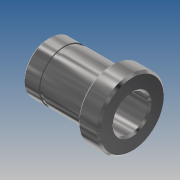
# Autodesk Inventor part: DD_KVD_004_03
Saved by Autodesk Inventor 2017.3 (Build 213256000, 256)
## iProperties
Created: 2012-08-17
Part Number: DD_KVD_004_03
Material: Nerezová ocel
Document SubType Name: Modeling
Designer: DAŘENA M.
Manufacturer: Standard
Standards Organization: Custom
Mass: 243.623 g
Surface Area: 187.558 cm^2
Volume: 30.4529 cm^3
Density: 8 g/cm^3
Appearance: Pololeštěná
HRUBA_HMOTNOST: 1,18 kg
POLOTOVAR_NORMA: ČSN 425510
ROZMER_POLOTOVARU: KR 80 - 30
Title: HRŘÍEL KLADKY
Author: DAŘENA M.
Autodesk Inventor part; units mm, degrees
ref_plane "YZ Plane" through (0, 0, 0) normal (1, 0, 0) x (0, 1, 0)
ref_plane "XZ Plane" through (0, 0, 0) normal (0, 1, 0) x (-1, 0, 0)
ref_plane "XY Plane" through (0, 0, 0) normal (0, 0, 1) x (1, 0, 0)
sketch "Náčrt1" plane through (0, 0, 0) normal (0, 0, 1) x (1, 0, 0)
  line L0 (-8, 0) -> (8, 0)
  line L1 (8, 0) -> (8, 27.5) construction
  line L2 (8, 27.5) -> (5.5, 27.5) construction
  line L3 (5.5, 27.5) -> (5.5, 26.5) construction
  line L4 (0.5, 21.5) -> (-0.5, 21.5) construction
  line L5 (-5.5, 26.5) -> (-5.5, 27.5) construction
  line L6 (-5.5, 27.5) -> (-8, 27.5) construction
  line L7 (-8, 27.5) -> (-8, 0) construction
  line L8 (-8, 16) -> (-6.85, 16) construction
  line L9 (-6.85, 16) -> (-6.85, 17.25) construction
  line L10 (-6.85, 17.25) -> (-5, 17.25) construction
  line L11 (-5, 17.25) -> (-5, 16) construction
  line L12 (-5, 16) -> (5, 16) construction
  line L13 (5, 16) -> (5, 14) construction
  line L14 (5, 14) -> (8, 14) construction
  arc A0 (-5.5, 26.5) -> (-0.5, 21.5) centre (-0.5, 26.5) ccw construction
  arc A1 (0.5, 21.5) -> (5.5, 26.5) centre (0.5, 26.5) ccw construction
  line L15 (5, 6) -> (5, 8)
  line L16 (5, 8) -> (10, 8)
  line L17 (10, 8) -> (10, 0)
  line L18 (10, 0) -> (8, 0)
  line L19 (-10, 6) -> (-10, 0)
  line L20 (-10, 0) -> (-8, 0)
  line L21 (-5, 6) -> (-5, 5.75)
  line L22 (-5, 5.75) -> (-6.1, 5.75)
  line L23 (-6.1, 5.75) -> (-6.1, 6)
  line L24 (-5, 6) -> (5, 6)
  line L25 (-6.1, 6) -> (-10, 6)
  point P0 (0, 0)
  point P1 (0, 0)
  point P2 (5.5, 21.5)
  point P3 (-5.5, 21.5)
  dimension "d0" = 55
  dimension "d1" = 16
  dimension "d3" = 2.5
  dimension "d4" = 6
  dimension "d5" = 32
  dimension "d6" = 28
  dimension "d7" = 10
  dimension "d8" = 13
  dimension "d9" = 34.5
  dimension "d10" = 1.85
  dimension "d18" = 11
  dimension "d24" = 43
  dimension "d27" = 5
  dimension "d31" = 16
  dimension "d32" = 2
  dimension "d33" = 2
  dimension "d34" = 1.1
  dimension "d35" = 11.5
  dimension "d36" = 12
  dimension "d37" = 20
  constraints: 52 end point, 10 horizontal, 9 vertical, 6 collinear, 6 perpendicular, 6 point on line, 4 point on circle, 4 tangent, 2 centre point, 2 coincident, 1 equal radius, 1 midpoint
  measures "d0" diameter of L1.end L0
  measures "d1" distance between parallel lines of L1 L7
  measures "d3" distance of L5.end L6.end
  measures "d4" distance of point (-5.5, 21.5) L5.end
  measures "d5" diameter of L12 L0
  measures "d6" diameter of L14 L0
  measures "d7" distance of L11.end L12.end
  measures "d8" distance from line of L7 L13.end
  measures "d9" diameter of L10 L0
  measures "d10" distance of L9.end L10.end
  measures "d18" distance of point (5.5, 21.5) point (-5.5, 21.5)
  measures "d24" diameter of L4 L0
  measures "d27" radius of A0
  measures "d31" diameter of L16 L0
  measures "d32" distance between parallel lines of L17 L1
  measures "d33" distance between parallel lines of L7 L19
  measures "d34" distance of L21.end L22.end
  measures "d35" diameter of L22 L0
  measures "d36" diameter of L25 L20
  measures "d37" distance between parallel lines of L17 L19
revolve "Rotace1" add sketch "Náčrt1" angle 360 about axis through (-8, 0, 0) along (1, 0, 0)
chamfer "Zkosení1" distance 0.5 angle 45 3 edges at (10, -8, 0) (-10, -6, 0) (5, -8, 0)
hole "Díra1" at (10, 0, 0) direction (-1, 0, 0) diameter 8.4 end through all clearance for "Strojní šroub se zápustnou hlavou" size "M8" standard "Ansi M metrický profil"
chamfer "Zkosení3" distance 0.4 angle 45 2 edges at (-10, 0, 4.2) (10, 0, 4.2)
